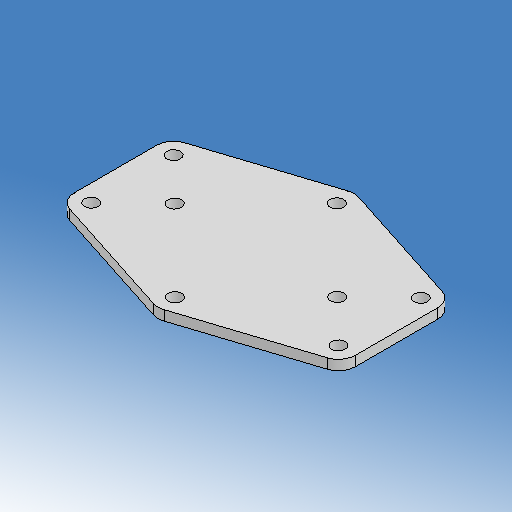
# Autodesk Inventor part: LidarMountAdapter
Saved by Autodesk Inventor 2025 (Build 290162000, 162)
## iProperties
Created: 2024-06-15
Part Number: LidarMountAdapter
Material: Generic
Document SubType Name: Sheet Metal
Designer: seene
Density: 1 g/cm^3
Sheet Metal Rule: Default
Appearance: Default
Author: seene
Autodesk Inventor part; units mm, degrees
ref_plane "YZ Plane" through (0, 0, 0) normal (1, 0, 0) x (0, 1, 0)
ref_plane "XZ Plane" through (0, 0, 0) normal (0, 1, 0) x (-1, 0, 0)
ref_plane "XY Plane" through (0, 0, 0) normal (0, 0, 1) x (1, 0, 0)
sketch "Sketch1" plane through (0, 0, 0) normal (0, 1, 0) x (-1, 0, 0)
  line L0 (-43.3451, -30.2749) -> (43.3451, -30.2749)
  line L1 (43.3451, -30.2749) -> (43.3451, 30.2749)
  line L2 (43.3451, 30.2749) -> (-43.3451, 30.2749)
  line L3 (-43.3451, 30.2749) -> (-43.3451, -30.2749)
  line L4 (-43.3451, -30.2749) -> (43.3451, 30.2749) construction
  line L5 (43.3451, -30.2749) -> (-43.3451, 30.2749) construction
  circle A0 centre (0, 0) radius 25 construction
  circle A1 centre (24.9999, 0.0535) radius 2.1
  circle A2 centre (-0.0535, 24.9999) radius 2.1
  circle A3 centre (-24.9999, -0.0535) radius 2.1
  circle A4 centre (0.0535, -24.9999) radius 2.1
  line L6 (25.4, -25.4) -> (-25.4, -25.4) construction
  line L7 (-25.4, -25.4) -> (-25.4, 25.4) construction
  line L8 (-25.4, 25.4) -> (25.4, 25.4) construction
  line L9 (25.4, 25.4) -> (25.4, -25.4) construction
  line L10 (25.4, -25.4) -> (-25.4, 25.4) construction
  line L11 (25.4, 25.4) -> (-25.4, -25.4) construction
  circle A5 centre (38.1, -12.7) radius 2.0701
  circle A6 centre (38.1, 12.7) radius 2.0701
  circle A7 centre (-38.1, 12.7) radius 2.0701
  circle A8 centre (-38.1, -12.7) radius 2.0701
  circle A9 centre (38.1, -12.7) radius 5.2451
  circle A10 centre (0.0535, -24.9999) radius 5.275
  circle A11 centre (-38.1, -12.7) radius 5.2451
  circle A12 centre (-0.0535, 24.9999) radius 5.275
  circle A13 centre (38.1, 12.7) radius 5.2451
  circle A14 centre (-38.1, 12.7) radius 5.2451
  line L12 (39.7131, 17.6909) -> (1.5688, 30.0193)
  line L13 (-1.6799, 30.018) -> (-39.7172, 17.6896)
  line L14 (-39.7131, -17.6909) -> (-1.5688, -30.0193)
  line L15 (39.7172, -17.6896) -> (1.6799, -30.018)
  point P0 (0, 0)
  point P1 (-43.3451, -12.7)
  point P2 (43.3451, -12.7)
  point P3 (43.3451, 12.7)
  point P4 (-43.3451, 12.7)
  dimension "d7" = 50
  dimension "d2" = 360
  dimension "d4" = 4.2
  dimension "d29" = 50.8
  dimension "d30" = 50.8
  dimension "d31" = 4.1402
  dimension "d32" = 4.1402
  dimension "d33" = 12.7
  dimension "d36" = 360
  dimension "d39" = 25.4
  dimension "d40" = 12.7
  dimension "d41" = 3.175
  dimension "d42" = 3.175
  dimension "d43" = 3.175
  dimension "d44" = 3.175
  dimension "d45" = 3.175
  dimension "d46" = 3.175
  measures "d4" diameter of A1
  measures "d29" distance of L7.end L8.end
  measures "d30" distance of L6.end L7.end
  measures "d31" diameter of A5
  measures "d32" diameter of A6
  measures "d33" distance from line of L9 A5.centre
  measures "d39" distance of A6.centre A5.centre
  measures "d40" vertical distance of point (0, 0) A5.centre
  measures "d42" radial gap between concentric circles of A4 A10
  measures "d44" radial gap between concentric circles of A2 A12
extrude "Plate1" add sketch "Sketch1" along normal blind 3.048 contours A10 | L3 A14 L13 A12 L12 A13 L1 A9 L15 A10 L14 A11 | A11 | A14 | A9 | A13 | A12
equation "\"d8\" = Thickness"
equation "\"d40\" = 0.5 * d39"
equation "\"BendRadius\" = Thickness"
equation "\"BendReliefWidth\" = Thickness"
equation "\"BendReliefDepth\" = 0.5 * Thickness"
equation "\"CornerReliefSize\" = 4 * Thickness"
equation "\"MinimumRemnant\" = 2 * Thickness"
equation "\"TransitionRadius\" = BendRadius"
equation "\"JacobiRadiusSize\" = BendRadius"
equation "\"GapSize\" = Thickness"
equation "\"Thickness\" = 3.048"
body "Solid1"
